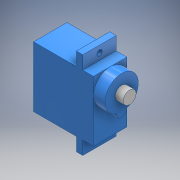
# Autodesk Inventor part: microservo
Saved by Autodesk Inventor 2018.3 (Build 223284000, 284)
## iProperties
Created: 2019-10-04
Part Number: microservo
Material: 一般
Document SubType Name: Modeling
Designer: Eiji Nishizawa
Density: 1 g/cm^3
Appearance: シアン
Author: Eiji Nishizawa
Autodesk Inventor part; units mm, degrees
ref_plane "YZ Plane" through (0, 0, 0) normal (1, 0, 0) x (0, 1, 0)
ref_plane "XZ Plane" through (0, 0, 0) normal (0, 1, 0) x (-1, 0, 0)
ref_plane "XY Plane" through (0, 0, 0) normal (0, 0, 1) x (1, 0, 0)
sketch "スケッチ1" plane through (0, 0, 0) normal (1, 0, 0) x (0, 1, 0)
  line L0 (6.25, 11.325) -> (-6.25, 11.325)
  line L1 (-6.25, 11.325) -> (-6.25, -11.325)
  line L2 (-6.25, -11.325) -> (6.25, -11.325)
  line L3 (6.25, -11.325) -> (6.25, 11.325)
  point P0 (0, 0)
  dimension "d0" = 22.65
  dimension "d1" = 12.5
  dimension "d4" = 6.25
  dimension "d5" = 6.25
  dimension "d6" = 11.325
  dimension "d7" = 11.325
  constraints: 8 end point, 2 parallel, 1 horizontal, 1 perpendicular
  measures "d0" distance of L2.end L0.start
  measures "d1" distance of L0.start L0.end
  measures "d4" distance from line of point (0, 0) L3
  measures "d5" distance from line of point (0, 0) L1
  measures "d6" distance from line of point (0, 0) L0
  measures "d7" distance from line of L2 point (0, 0)
extrude "押し出し1" add sketch "スケッチ1" along normal blind 16
sketch "スケッチ2" plane through (16, 0, 0) normal (1, 0, 0) x (0, 0, -1)
  line L0 (-11.325, 6.25) -> (-11.325, -6.25) projected
  line L1 (-11.325, 6.25) -> (-16.325, 6.25)
  line L2 (-16.325, 6.25) -> (-16.325, -6.25)
  line L3 (-16.325, -6.25) -> (-11.325, -6.25)
  line L4 (-11.325, -6.25) -> (-11.325, 6.25)
  line L5 (11.325, -6.25) -> (11.325, 6.25) projected
  line L6 (11.325, 6.25) -> (16.325, 6.25)
  line L7 (16.325, 6.25) -> (16.325, -6.25)
  line L8 (16.325, -6.25) -> (11.325, -6.25)
  line L9 (11.325, -6.25) -> (11.325, 6.25)
  circle A0 centre (-13.825, 0) radius 1
  circle A1 centre (13.825, 0) radius 1
  line L10 (-11.325, -6.25) -> (11.325, -6.25) projected
  line L11 (-11.325, 6.25) -> (11.325, 6.25)
  line L12 (11.325, 6.25) -> (11.325, -6.25)
  line L13 (11.325, -6.25) -> (-11.325, -6.25)
  line L14 (-11.325, -6.25) -> (-11.325, 6.25)
  point P0 (0, 0)
  dimension "d8" = 5
  dimension "d9" = 5
  dimension "d10" = 1.5
  dimension "d11" = 1.5
  dimension "d12" = 2
  dimension "d13" = 2
  constraints: 24 end point, 6 parallel, 3 horizontal, 3 perpendicular, 2 centre point, 1 point on line
  measures "d8" distance between parallel lines of L0 L2
  measures "d9" distance between parallel lines of L5 L7
  measures "d10" distance edge to line of A0 L2
  measures "d11" distance edge to line of A1 L7
  measures "d12" diameter of A1
  measures "d13" diameter of A0
extrude "押し出し2" add sketch "スケッチ2" along normal blind 2.4
sketch "スケッチ3" plane through (18.4, 0, 0) normal (1, 0, 0) x (0, 0, -1)
  line L0 (-11.325, 6.25) -> (-11.325, -6.25) projected
  line L1 (11.325, -6.25) -> (16.325, -6.25) projected
  line L2 (-11.325, 6.25) -> (11.325, 6.25)
  line L3 (11.325, 6.25) -> (11.325, -6.25)
  line L4 (11.325, -6.25) -> (-11.325, -6.25)
  line L5 (-11.325, -6.25) -> (-11.325, 6.25)
  point P0 (0, 0)
  constraints: 8 end point, 2 parallel, 1 horizontal, 1 perpendicular
extrude "押し出し3" add sketch "スケッチ3" along normal blind 4
sketch "スケッチ4" plane through (22.4, 0, 0) normal (1, 0, 0) x (0, 0, -1)
  circle A0 centre (-5.0802, 0) radius 6.2448
  line L0 (-11.325, 6.25) -> (-11.325, -6.25) projected
  circle A1 centre (1.0094, 0) radius 1.9656
  circle A2 centre (-5.0802, 0) radius 2.4
  point P0 (0, 0)
  dimension "d18" = 0
  dimension "d19" = 12.4895
  dimension "d20" = 3.9311
  dimension "d21" = 14.3
  dimension "d22" = 4.8
  constraints: 3 centre point, 1 coincident
  measures "d18" distance edge to line of A0 L0
  measures "d19" diameter of A0
  measures "d20" diameter of A1
  measures "d22" diameter of A2
extrude "押し出し4" add sketch "スケッチ4" along normal blind 4.3
sketch "スケッチ5" plane through (22.4, 0, 5.0802) normal (1, 0, 0) x (0, 0, -1)
  circle A0 centre (0, 0) radius 2.4
  point P0 (5.0802, 0)
  constraints: 1 centre point
extrude "押し出し5" add sketch "スケッチ5" along normal blind 7.3
